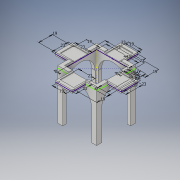
# Autodesk Inventor part: Holder_ArUco_4_Markers
Saved by Autodesk Inventor 2019 (Build 230136000, 136)
## iProperties
Created: 2019-03-16
Part Number: Holder_ArUco_4_Markers
Material: Generic
Document SubType Name: Modeling
Designer: vah12
Density: 1 g/cm^3
Appearance: Default
Author: vah12
## iProperties of the stored document Holder_ArUco_4_Markers_3DPrint.ipt
Created: 2019-03-17
Part Number: Holder_ArUco_4_Markers_3DPrint
Material: Generic
Document SubType Name: Modeling
Designer: vah12
Density: 1 g/cm^3
Appearance: Default
Author: vah12
Autodesk Inventor part; units mm, degrees
ref_plane "YZ Plane" through (0, 0, 0) normal (1, 0, 0) x (0, 1, 0)
ref_plane "XZ Plane" through (0, 0, 0) normal (0, 1, 0) x (-1, 0, 0)
ref_plane "XY Plane" through (0, 0, 0) normal (0, 0, 1) x (1, 0, 0)
sketch "Sketch1" plane through (0, 0, 0) normal (0, 1, 0) x (-1, 0, 0)
  line L0 (22.25, 22.25) -> (-22.25, 22.25)
  line L1 (-22.25, 22.25) -> (-22.25, -22.25)
  line L2 (-22.25, -22.25) -> (22.25, -22.25)
  line L3 (22.25, -22.25) -> (22.25, 22.25)
  line L4 (22.25, 22.25) -> (-22.25, -22.25) construction
  line L5 (-22.25, 22.25) -> (22.25, -22.25) construction
  line L6 (27, 27) -> (-27, 27)
  line L7 (-27, 27) -> (-27, -27)
  line L8 (-27, -27) -> (27, -27)
  line L9 (27, -27) -> (27, 27)
  line L10 (27, 27) -> (-27, -27) construction
  line L11 (-27, 27) -> (27, -27) construction
  line L12 (11.5, 22.25) -> (-11.5, 22.25)
  line L13 (-11.5, 22.25) -> (-11.5, 45.25)
  line L14 (-11.5, 45.25) -> (11.5, 45.25)
  line L15 (11.5, 45.25) -> (11.5, 22.25)
  line L16 (11.5, 22.25) -> (-11.5, 45.25) construction
  line L17 (-11.5, 22.25) -> (11.5, 45.25) construction
  line L18 (-9.5, 41.25) -> (9.5, 41.25)
  line L19 (9.5, 41.25) -> (9.5, 22.25)
  line L20 (9.5, 22.25) -> (-9.5, 22.25)
  line L21 (-9.5, 22.25) -> (-9.5, 41.25)
  line L22 (-9.5, 41.25) -> (9.5, 22.25) construction
  line L23 (9.5, 41.25) -> (-9.5, 22.25) construction
  line L24 (45.25, 11.5) -> (22.25, 11.5)
  line L25 (22.25, 11.5) -> (22.25, -11.5)
  line L26 (22.25, -11.5) -> (45.25, -11.5)
  line L27 (45.25, -11.5) -> (45.25, 11.5)
  line L28 (45.25, 11.5) -> (22.25, -11.5) construction
  line L29 (22.25, 11.5) -> (45.25, -11.5) construction
  line L30 (22.25, 9.5) -> (41.25, 9.5)
  line L31 (41.25, 9.5) -> (41.25, -9.5)
  line L32 (41.25, -9.5) -> (22.25, -9.5)
  line L33 (22.25, -9.5) -> (22.25, 9.5)
  line L34 (22.25, 9.5) -> (41.25, -9.5) construction
  line L35 (41.25, 9.5) -> (22.25, -9.5) construction
  line L36 (-11.5, -22.25) -> (11.5, -22.25)
  line L37 (11.5, -22.25) -> (11.5, -45.25)
  line L38 (11.5, -45.25) -> (-11.5, -45.25)
  line L39 (-11.5, -45.25) -> (-11.5, -22.25)
  line L40 (-11.5, -22.25) -> (11.5, -45.25) construction
  line L41 (11.5, -22.25) -> (-11.5, -45.25) construction
  line L42 (-9.5, -22.25) -> (9.5, -22.25)
  line L43 (9.5, -22.25) -> (9.5, -41.25)
  line L44 (9.5, -41.25) -> (-9.5, -41.25)
  line L45 (-9.5, -41.25) -> (-9.5, -22.25)
  line L46 (-9.5, -22.25) -> (9.5, -41.25) construction
  line L47 (9.5, -22.25) -> (-9.5, -41.25) construction
  line L48 (-45.25, 11.5) -> (-22.25, 11.5)
  line L49 (-22.25, 11.5) -> (-22.25, -11.5)
  line L50 (-22.25, -11.5) -> (-45.25, -11.5)
  line L51 (-45.25, -11.5) -> (-45.25, 11.5)
  line L52 (-45.25, 11.5) -> (-22.25, -11.5) construction
  line L53 (-22.25, 11.5) -> (-45.25, -11.5) construction
  line L54 (-41.25, 9.5) -> (-22.25, 9.5)
  line L55 (-22.25, 9.5) -> (-22.25, -9.5)
  line L56 (-22.25, -9.5) -> (-41.25, -9.5)
  line L57 (-41.25, -9.5) -> (-41.25, 9.5)
  line L58 (-41.25, 9.5) -> (-22.25, -9.5) construction
  line L59 (-22.25, 9.5) -> (-41.25, -9.5) construction
  point P0 (0, 0)
  point P1 (0, 33.75)
  point P2 (0, 31.75)
  point P3 (0, 22.25)
  point P4 (33.75, 0)
  point P5 (31.75, 0)
  point P6 (0, -33.75)
  point P7 (0, -31.75)
  point P8 (-33.75, 0)
  point P9 (-31.75, 0)
  point P10 (-22.25, 0)
  point P11 (0, -22.25)
  point P12 (31.75, 0)
  point P13 (33.75, 0)
  point P14 (22.25, 0)
  point P15 (0, -31.75)
  point P16 (0, -33.75)
  point P17 (-31.75, 0)
  point P18 (-33.75, 0)
  point P19 (0, 31.75)
  point P20 (0, 33.75)
  dimension "d0" = 44.5
  dimension "d1" = 44.5
  dimension "d2" = 54
  dimension "d3" = 54
  dimension "d55" = 23
  dimension "d56" = 23
  dimension "d67" = 0
  dimension "d68" = 19
  dimension "d69" = 19
  dimension "d70" = 23
  dimension "d71" = 23
  dimension "d72" = 19
  dimension "d73" = 19
  dimension "d74" = 0
  dimension "d75" = 23
  dimension "d76" = 23
  dimension "d77" = 19
  dimension "d78" = 0
  dimension "d79" = 19
  dimension "d80" = 23
  dimension "d81" = 23
  dimension "d82" = 19
  dimension "d83" = 19
  dimension "d84" = 0
  constraints: 120 end point, 36 midpoint, 19 parallel, 10 horizontal, 10 perpendicular, 2 horizontal alignment, 2 vertical alignment, 1 point on line
  measures "d0" distance of L1.end L2.end
  measures "d1" distance of L0.end L1.end
  measures "d2" distance of L7.end L8.end
  measures "d3" distance of L6.end L7.end
  measures "d55" distance of L12.end L14.start
  measures "d56" distance of L12.start L12.end
  measures "d67" distance between parallel lines of L20 L12
  measures "d68" distance of L20.end L18.start
  measures "d69" distance of L18.start L18.end
  measures "d70" distance of L25.end L26.end
  measures "d71" distance of L26.end L24.start
  measures "d72" distance of L31.end L32.end
  measures "d73" distance of L30.end L31.end
  measures "d74" distance between parallel lines of L33 L25
  measures "d75" distance of L38.end L36.start
  measures "d76" distance of L37.end L38.end
  measures "d77" distance of L43.end L44.end
  measures "d78" distance between parallel lines of L2 L42
  measures "d79" distance of L44.end L42.start
  measures "d80" distance of L49.end L50.end
  measures "d81" distance of L50.end L48.start
  measures "d82" distance of L56.end L54.start
  measures "d83" distance of L55.end L56.end
  measures "d84" distance between parallel lines of L1 L55
extrude "Extrusion1" add sketch "Sketch1" against normal blind 66 contours L0 L15 L6 L9 L24 L3 | L0 L19 L6 L15 | L24 L9 L30 L3 | L0 L21 L6 L19 | L30 L9 L32 L3 | L0 L13 L6 L21 | L32 L9 L26 L3 | L0 L1 L48 L7 L6 L13 | L26 L9 L8 L37 L2 L3 | L1 L54 L7 L48 | L37 L8 L43 L2 | L1 L56 L7 L54 | L43 L8 L45 L2 | L1 L50 L7 L56 | L45 L8 L39 L2 | L1 L2 L39 L8 L7 L50
sketch "Sketch3" plane through (-27, -66, 27) normal (0, 0, 1) x (1, 0, 0)
  line L0 (0, 66) -> (0, 0) projected
  line L1 (54, 0) -> (0, 0) projected
  line L2 (54, 66) -> (54, 0) projected
  arc A0 (47, 42) -> (7, 42) centre (27, 42) ccw
  line L3 (38.5, 62) -> (15.5, 62) projected
  line L4 (7, 42) -> (7, 0)
  line L5 (54, 0) -> (0, 0) projected
  line L6 (47, 42) -> (47, 0)
  line L7 (0, 66) -> (54, 66) projected
  point P0 (27, 66)
  point P1 (27, 62)
  dimension "d42" = 20
  constraints: 4 end point, 3 point on circle, 2 point on line, 1 centre point, 1 midpoint, 1 perpendicular, 1 tangent, 1 vertical
  measures "d42" radius of A0
extrude "Extrusion5" cut sketch "Sketch3" against normal through all contours L4 A0 L6 L1
sketch "Sketch4" plane through (27, -66, 27) normal (1, 0, 0) x (0, 0, -1)
  line L0 (0, 66) -> (0, 0) projected
  line L1 (54, 0) -> (0, 0) projected
  line L2 (54, 66) -> (54, 0) projected
  line L3 (38.5, 62) -> (15.5, 62) projected
  arc A0 (47, 42) -> (7, 42) centre (27, 42) ccw
  line L4 (7, 42) -> (7, 0)
  line L5 (47, 42) -> (47, 0)
  line L6 (54, 0) -> (0, 0) projected
  line L7 (0, 66) -> (54, 66) projected
  point P0 (27, 66)
  point P1 (27, 62)
  dimension "d46" = 20
  constraints: 4 end point, 3 point on circle, 2 point on line, 1 centre point, 1 midpoint, 1 perpendicular, 1 tangent, 1 vertical
  measures "d46" radius of A0
extrude "Extrusion6" cut sketch "Sketch4" against normal through all contours L4 A0 L5 L1
extrude "Extrusion7" add sketch "Sketch1" along normal mid plane 4 contours L0 L19 L6 L15 | L24 L9 L30 L3 | L6 L19 L18 L21 L13 L14 L15 | L24 L27 L26 L9 L32 L31 L30 | L0 L13 L6 L21 | L32 L9 L26 L3 | L1 L54 L7 L48 | L37 L8 L43 L2 | L7 L54 L57 L56 L50 L51 L48 | L37 L38 L39 L8 L45 L44 L43 | L1 L50 L7 L56 | L45 L8 L39 L2
extrude "Extrusion8" add sketch "Sketch1" along normal blind 1 and the other way blind 2 contours L0 L21 L6 L19 | L30 L9 L32 L3 | L6 L21 L18 L19 | L30 L31 L32 L9 | L1 L56 L7 L54 | L43 L8 L45 L2 | L7 L56 L57 L54 | L43 L44 L45 L8
sketch "Sketch5" plane through (0, 0, 0) normal (0, 1, 0) x (1, 0, 0)
  line L0 (-11.5, -27) -> (-11.5, -22.25) projected
  line L1 (-11.5, -22.25) -> (-22.25, -22.25) projected
  line L2 (-22.25, -22.25) -> (-22.25, -11.5) projected
  line L3 (-22.25, -11.5) -> (-27, -11.5) projected
  line L4 (-27, -11.5) -> (-27, -27) projected
  line L5 (-27, -27) -> (-11.5, -27) projected
  line L6 (-27, 11.5) -> (-22.25, 11.5) projected
  line L7 (-22.25, 11.5) -> (-22.25, 22.25) projected
  line L8 (-22.25, 22.25) -> (-11.5, 22.25) projected
  line L9 (-11.5, 22.25) -> (-11.5, 27) projected
  line L10 (-11.5, 27) -> (-27, 27) projected
  line L11 (-27, 27) -> (-27, 11.5) projected
  line L12 (22.25, 11.5) -> (27, 11.5) projected
  line L13 (27, 11.5) -> (27, 27) projected
  line L14 (27, 27) -> (11.5, 27) projected
  line L15 (11.5, 27) -> (11.5, 22.25) projected
  line L16 (11.5, 22.25) -> (22.25, 22.25) projected
  line L17 (22.25, 22.25) -> (22.25, 11.5) projected
  line L18 (27, -11.5) -> (22.25, -11.5) projected
  line L19 (22.25, -11.5) -> (22.25, -22.25) projected
  line L20 (22.25, -22.25) -> (11.5, -22.25) projected
  line L21 (11.5, -22.25) -> (11.5, -27) projected
  line L22 (11.5, -27) -> (27, -27) projected
  line L23 (27, -27) -> (27, -11.5) projected
  point P0 (0, 0)
extrude "Extrusion9" add sketch "Sketch5" along normal blind 3
body "Solid1"
